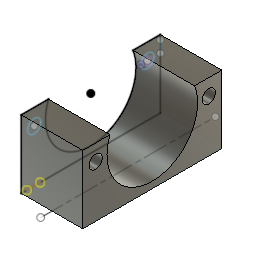
MOTOR-MOUNT (Autodesk Fusion 360 design; units mm, degrees)
Autodesk Fusion 360 part; units mm, degrees
sketch "Sketch1" plane through (0, 0, 0) normal (1, 0, 0) x (0, 1, 0)
  line L0 (21.5, 5) -> (21.5, -16)
  line L1 (21.5, -16) -> (-21.5, -16)
  line L2 (-21.5, -16) -> (-21.5, 5)
  line L3 (-21.5, 5) -> (-13.0767, 5)
  line L4 (13.0767, 5) -> (21.5, 5)
  arc A0 (-13.0767, 5) -> (13.0767, 5) centre (0, 0) ccw
  circle A1 centre (17.5, -0.0047) radius 2.05
  circle A2 centre (-17.5, 0) radius 2.05
  dimension "d44" = 28
  dimension "d47" = 16
  dimension "d48" = 5
  dimension "d49" = 4.1
  dimension "d50" = 21.5
  dimension "d51" = 21.5
  dimension "d52" = 17.5
  dimension "d56" = 4.1
  dimension "d57" = 17.5
  constraint coincident A0.centre origin
  constraint horizontal L3
  constraint vertical L0
  constraint horizontal L1
  constraint vertical L2
  constraint collinear L3 L4
  measures "d44" diameter of A0
  measures "d47" distance of A0.centre L1
  measures "d48" distance of A0.centre L4
  measures "d49" diameter of A1
  measures "d50" distance of A0.centre L0
  measures "d51" horizontal distance of A0.centre L2.end
  measures "d52" horizontal distance of A0.centre A1.centre
  measures "d56" diameter of A2
  measures "d57" distance of A0.centre A2.centre
extrude "Extrude1" add sketch "Sketch1" along normal blind 19
sketch "Sketch2" plane through (0, 0, 0) normal (1, 0, 0) x (0, 1, 0)
  line L0 (21.5, 3.5453) -> (21.5, -0.0047)
  point P0 (15.45, -0.0047)
  point P1 (17.5, -0.0047)
  dimension "d62" = 4
  measures "d62" distance of L0 P1
sketch "Sketch3" plane through (0, 0, -16) normal (0, 0, -1) x (1, 0, 0)
  line L0 (0, 21.5) -> (0, -21.5)
  line L1 (0, -21.5) -> (19, -21.5)
  line L2 (19, -21.5) -> (19, 21.5)
  line L3 (19, 21.5) -> (0, 21.5)
  line L4 (9.5, 25) -> (9.5, -29)
  dimension "d63" = 9.5
  constraint perpendicular L1 L4
  measures "d63" horizontal distance of origin L4.start
sketch "Sketch4" plane through (0, 0, -16) normal (0, 0, -1) x (1, 0, 0)
sketch "Sketch5" plane through (0, 0, 0) normal (1, 0, 0) x (0, 1, 0)
  line L0 (-19.794, -16) -> (-15.6772, -16)
  dimension "d64" = 4.1168
  dimension "d65" = 4.1168
  measures "d64" distance of L0.start L0.end
  measures "d65" distance of L0.start L0.end
sketch "Sketch6" plane through (0, 0, -16) normal (0, 0, -1) x (1, 0, 0)
  circle A0 centre (9.5, 18) radius 1
  line L0 (19, 21.5) -> (0, 21.5)
  circle A1 centre (9.5, -18) radius 1
  line L1 (0, -21.5) -> (19, -21.5)
  dimension "d66" = 2
  dimension "d67" = 3.5
  dimension "d68" = 2
  dimension "d69" = 3.5
  measures "d66" diameter of A0
  measures "d67" distance of A0.centre L0
  measures "d68" diameter of A1
  measures "d69" distance of A1.centre L1
extrude "Extrude2" cut sketch "Sketch6" against normal blind 10
